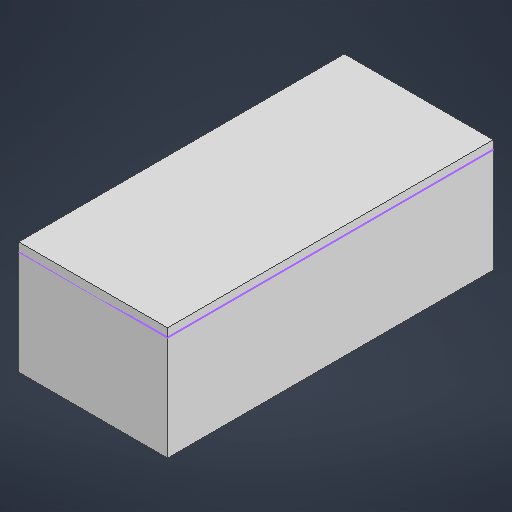
# Autodesk Inventor part: Part1
Saved by Autodesk Inventor 2026.2 (Build 302298010, 298A)
## iProperties
Created: 2026-03-25
Part Number: Part1
Material: Generic
Document SubType Name: Modeling
Designer: Srishanth Dhondy
Density: 1 g/cm^3
Appearance: Default
Author: Srishanth Dhondy
Autodesk Inventor part; units mm, degrees
ref_plane "YZ Plane" through (0, 0, 0) normal (1, 0, 0) x (0, 1, 0)
ref_plane "XZ Plane" through (0, 0, 0) normal (0, 1, 0) x (-1, 0, 0)
ref_plane "XY Plane" through (0, 0, 0) normal (0, 0, 1) x (1, 0, 0)
sketch "Sketch1" plane through (0, 0, 0) normal (0, 1, 0) x (-1, 0, 0)
  line L0 (-6.5941, -14.4299) -> (6.5941, -14.4299)
  line L1 (6.5941, -14.4299) -> (6.5941, 14.4299)
  line L2 (6.5941, 14.4299) -> (-6.5941, 14.4299)
  line L3 (-6.5941, 14.4299) -> (-6.5941, -14.4299)
  line L4 (-6.5941, -14.4299) -> (6.5941, 14.4299) construction
  line L5 (6.5941, -14.4299) -> (-6.5941, 14.4299) construction
  line L6 (-5.5833, -13.4191) -> (5.5833, -13.4191)
  line L7 (5.5833, -13.4191) -> (5.5833, 13.4191)
  line L8 (5.5833, 13.4191) -> (-5.5833, 13.4191)
  line L9 (-5.5833, 13.4191) -> (-5.5833, -13.4191)
  point P0 (0, 0)
  constraints: 20 end point, 4 parallel, 2 midpoint, 2 perpendicular, 1 horizontal, 3 other
extrude "Extrusion1" add sketch "Sketch1" along normal blind 0.75 contours L3 L2 L1 L0 | L9 L8 L7 L6
extrude "Extrusion2" add sketch "Sketch1" against normal blind 9.25
body "Solid1"
